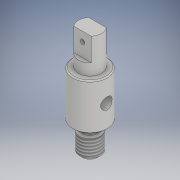
# Autodesk Inventor part: Вал_19
Saved by Autodesk Inventor 2019.3 (Build 233278000, 278)
## iProperties
Created: 2020-04-04
Part Number: Вал_19
Material: Типовые
Document SubType Name: Modeling
Designer: Пользователь
Density: 1 g/cm^3
Appearance: По умолчанию
Author: Пользователь
Autodesk Inventor part; units mm, degrees
ref_plane "XZ Plane" through (0, 0, 0) normal (0, 1, 0) x (-1, 0, 0)
ref_plane "XY Plane" through (0, 0, 0) normal (0, 0, 1) x (1, 0, 0)
sketch "Эскиз1" plane through (0, 0, 0) normal (1, 0, 0) x (0, 1, 0)
  line L0 (0, 0) -> (0, 9)
  line L1 (0, 9) -> (17.25, 9)
  line L2 (17.25, 9) -> (18.7071, 7.5429)
  line L3 (19.4142, 7.25) -> (23.4, 7.25)
  line L4 (25, 8.85) -> (25, 15)
  line L5 (25, 15) -> (65, 15)
  line L6 (65, 15) -> (65, 10)
  line L7 (65, 10) -> (95, 10)
  line L8 (95, 0) -> (0, 0)
  line L9 (95, 10) -> (95, 0)
  arc A0 (18.7071, 7.5429) -> (19.4142, 7.25) centre (19.4142, 8.25) ccw
  arc A1 (23.4, 7.25) -> (25, 8.85) centre (23.4, 8.85) ccw
  point P0 (19, 7.25)
  point P1 (25, 7.25)
  dimension "d0" = 95
  dimension "d1" = 18
  dimension "d2" = 14.5
  dimension "d3" = 45
  dimension "d4" = 40
  dimension "d5" = 25
  dimension "d6" = 6
  dimension "d7" = 20
  dimension "d8" = 30
  dimension "d9" = 1
  dimension "d10" = 1.6
  constraints: 20 end point, 4 horizontal, 4 point on circle, 4 point on line, 4 tangent, 4 vertical, 2 centre point, 1 coincident, 1 horizontal alignment
  measures "d0" distance of L8.start point (0, 0)
  measures "d1" diameter of L1 L8
  measures "d2" diameter of L3 L8
  measures "d3" angle of L1 L2
  measures "d4" distance between parallel lines of L6 L4
  measures "d5" distance between parallel lines of L0 L4
  measures "d6" distance of point (25, 7.25) point (19, 7.25)
  measures "d7" diameter of L7 L8
  measures "d8" diameter of L5 L8
  measures "d9" radius of A0
  measures "d10" radius of A1
revolve "Вращение1" add sketch "Эскиз1" angle 360 about axis through (0, 95, 0) along (0, -1, 0)
thread "Резьба1" size "M18x2.5" designation "M18" class "6g" standard "GB Metric profile" full length
chamfer "Фаска1" distance 2.5 angle 45 1 edges at (0, 0, -9)
chamfer "Фаска2" distance 1 angle 45 2 edges at (0, 25, -15) (0, 65, -15)
ref_plane "РабПлоскость1" through (15, 0, 0) normal (1, 0, 0) x (0, 1, 0)
sketch "Эскиз2" plane through (15, 0, 0) normal (1, 0, 0) x (0, 1, 0)
  line L0 (25, -14) -> (25, 14) projected
  point P0 (0, 0)
  point P1 (45, 0)
  dimension "d21" = 20
  constraints: 1 horizontal alignment
  measures "d21" distance from line of L0 point (45, 0)
hole "Отверстие1" at (15, 45, 0) direction (-1, 0, 0) diameter 10 depth 15 tip angle 120
sketch "Эскиз3" plane through (0, 0, 0) normal (1, 0, 0) x (0, 1, 0)
  line L0 (95, 10) -> (75, 10)
  line L1 (75, 10) -> (75, 6.5)
  line L2 (75, 6.5) -> (95, 6.5)
  line L3 (95, 6.5) -> (95, 10)
  line L4 (-19.7495, 0) -> (118.4967, 0) projected
  line L5 (95, -10) -> (95, 10) projected
  line L6 (65, 10) -> (95, 10) projected
  line L7 (-19, 0) -> (114, 0) projected
  line L8 (95, -10) -> (75, -10)
  line L9 (75, -10) -> (75, -6.5)
  line L10 (75, -6.5) -> (95, -6.5)
  line L11 (95, -6.5) -> (95, -10)
  point P0 (0, 0)
  dimension "d29" = 6.5
  dimension "d30" = 20
  constraints: 16 end point, 6 symmetric about line, 2 horizontal, 2 point on line, 2 vertical
  measures "d29" distance between parallel lines of L4 L2
  measures "d30" distance between parallel lines of L1 L3
extrude "Выдавливание1" cut sketch "Эскиз3" along normal through all both and the other way through all
sketch "Эскиз4" plane through (-7.5993, 95, 6.5) normal (0, 0, 1) x (1, 0, 0)
  line L0 (0, 0) -> (15.1987, 0) projected
  line L1 (-2.4007, -30) -> (-2.4007, 0) projected
  point P0 (7.5993, -95)
  point P1 (7.5993, -8)
  dimension "d33" = 10
  dimension "d34" = 8
  measures "d33" distance from line of L1 point (7.599, -8)
  measures "d34" distance from line of L0 point (7.599, -8)
hole "Отверстие2" at (0, 87, 6.5) direction (0, 0, -1) diameter 4 end through all
